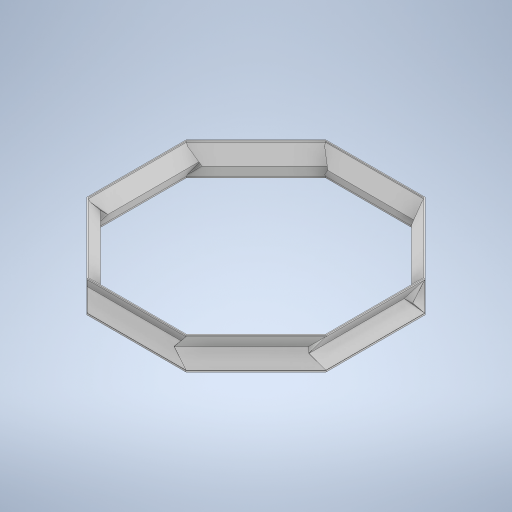
# Autodesk Inventor part: 팔각형 OV-PAM 층 한개
Saved by Autodesk Inventor 2024 (Build 280153000, 153)
## iProperties
Created: 2023-06-16
Part Number: 팔각형 OV-PAM 층 한개
Material: 일반
Document SubType Name: Modeling
Designer: jsw
Density: 1 g/cm^3
Appearance: 기본값
Author: jsw
Autodesk Inventor part; units mm, degrees
ref_plane "YZ Plane" through (0, 0, 0) normal (1, 0, 0) x (0, 1, 0)
ref_plane "XZ Plane" through (0, 0, 0) normal (0, 1, 0) x (-1, 0, 0)
ref_plane "XY Plane" through (0, 0, 0) normal (0, 0, 1) x (1, 0, 0)
sketch "스케치1" plane through (0, 0, 0) normal (0, 1, 0) x (-1, 0, 0)
  line L0 (-97.7756, 40.5) -> (-40.5, 97.7756)
  line L1 (-40.5, 97.7756) -> (40.5, 97.7756)
  line L2 (40.5, 97.7756) -> (97.7756, 40.5)
  line L3 (97.7756, 40.5) -> (97.7756, -40.5)
  line L4 (97.7756, -40.5) -> (40.5, -97.7756)
  line L5 (40.5, -97.7756) -> (-40.5, -97.7756)
  line L6 (-40.5, -97.7756) -> (-97.7756, -40.5)
  line L7 (-97.7756, -40.5) -> (-97.7756, 40.5)
  line L8 (-40.7485, 98.3756) -> (40.7485, 98.3756)
  line L9 (40.7485, 98.3756) -> (98.3756, 40.7485)
  line L10 (98.3756, 40.7485) -> (98.3756, -40.7485)
  line L11 (98.3756, -40.7485) -> (40.7485, -98.3756)
  line L12 (40.7485, -98.3756) -> (-40.7485, -98.3756)
  line L13 (-40.7485, -98.3756) -> (-98.3756, -40.7485)
  line L14 (-98.3756, -40.7485) -> (-98.3756, 40.7485)
  line L15 (-98.3756, 40.7485) -> (-40.7485, 98.3756)
  point P0 (0, 0)
  point P1 (0, 0)
  point P2 (0, 0)
  dimension "d0" = 81
  dimension "d2" = 0.6
  constraints: 32 end point, 2 coincident, 2 horizontal, 34 other
  measures "d0" distance of L0.end L1.end
  measures "d2" distance between parallel lines of L10 L3
extrude "돌출2" add sketch "스케치1" along normal blind 12 contours L0 L1 L2 L3 L4 L5 L6 L7 | L8 L9 L10 L11 L12 L13 L14 L15
ref_plane "작업 평면2" through (98.3756, 0, 40.7485) normal (-0.8660254, -0.5, 0) x (0, 0, -1)
sketch "스케치3" plane through (98.3756, 0, 40.7485) normal (1, 0, 0) x (0, 0, -1)
  line L0 (0, 0) -> (0, 12) projected
  line L1 (0, 12) -> (81.4971, 12) projected
  line L2 (0, 0) -> (81.4971, 0)
  line L3 (81.4971, 0) -> (81.4971, 12)
  line L4 (81.4971, 12) -> (0, 12)
  line L5 (0, 12) -> (0, 0)
  line L6 (0, 12) -> (-7.3047, 12)
  line L7 (-57.6271, 12) -> (0, 12) projected
  line L8 (0, 0) -> (-7.3047, 12)
  line L9 (81.4971, 12) -> (40.7485, 12)
  line L10 (71.4971, 12) -> (81.4971, 0)
  point P0 (40.7485, 0)
  point P1 (71.4971, 12)
  point P2 (40.7485, 12)
  dimension "d17" = 121.33
  dimension "d53" = 10
  constraints: 16 end point, 5 midpoint, 2 parallel, 2 point on line, 1 horizontal, 1 perpendicular
  measures "d17" angle of L8 L2
  measures "d53" distance of L1.end L10.start
extrude "돌출4" cut sketch "스케치3" against normal up to surface contours L8 L6 L0 | L0 L1 L10 L2 surface through (98.3756, 0, 40.7485) normal (-0.8660254, -0.5, 0)
pattern_circular "원형 패턴1" count 8 over 360 about axis through (0, -10, 0) along (0, 1, 0) of "돌출4"
mirror "미러5" about plane through (0, 12, 0) normal (0, 1, 0) of "돌출2", "돌출4", "원형 패턴1"
sketch "스케치9" plane through (-40.7485, 24, -98.3756) normal (0, 1, 0) x (1, 0, 0)
  line L0 (139.1242, -139.1242) -> (139.1242, -57.6271) projected
  line L1 (139.1242, -57.6271) -> (81.4971, 0) projected
  line L2 (81.4971, 0) -> (0, 0) projected
  line L3 (0, 0) -> (-57.6271, -57.6271) projected
  line L4 (-57.6271, -57.6271) -> (-57.6271, -139.1242) projected
  line L5 (-57.6271, -139.1242) -> (0, -196.7513) projected
  line L6 (0, -196.7513) -> (81.4971, -196.7513) projected
  line L7 (81.4971, -196.7513) -> (139.1242, -139.1242) projected
  point P0 (40.7485, -98.3756)
extrude "돌출8" add sketch "스케치9" along normal blind 1.2
sketch "스케치10" plane through (0, 0, 0) normal (0, -1, 0) x (1, 0, 0)
  line L0 (98.3756, 40.7485) -> (98.3756, -40.7485) projected
  line L1 (40.7485, 98.3756) -> (98.3756, 40.7485) projected
  line L2 (-40.7485, 98.3756) -> (40.7485, 98.3756) projected
  line L3 (-98.3756, 40.7485) -> (-40.7485, 98.3756) projected
  line L4 (-98.3756, -40.7485) -> (-98.3756, 40.7485) projected
  line L5 (-40.7485, -98.3756) -> (-98.3756, -40.7485) projected
  line L6 (40.7485, -98.3756) -> (-40.7485, -98.3756) projected
  line L7 (98.3756, -40.7485) -> (40.7485, -98.3756) projected
  point P0 (0, 0)
extrude "돌출9" add sketch "스케치10" along normal blind 1.2
shell "쉘6" thickness 0.6 removed faces 2 at (-13.5828, 25.2, 32.7919) at (13.5828, -1.2, 32.7919)
sketch "스케치12" plane through (-40.7485, 25.2, -98.3756) normal (0, 1, 0) x (1, 0, 0)
  line L0 (138.5242, -57.8756) -> (138.5242, -138.8756) projected
  line L1 (138.5242, -138.8756) -> (81.2485, -196.1513) projected
  line L2 (81.2485, -196.1513) -> (0.2485, -196.1513) projected
  line L3 (0.2485, -196.1513) -> (-57.0271, -138.8756) projected
  line L4 (-57.0271, -138.8756) -> (-57.0271, -57.8756) projected
  line L5 (-57.0271, -57.8756) -> (0.2485, -0.6) projected
  line L6 (0.2485, -0.6) -> (81.2485, -0.6) projected
  line L7 (81.2485, -0.6) -> (138.5242, -57.8756) projected
  line L8 (139.1242, -57.6271) -> (81.4971, 0) projected
  line L9 (81.4971, 0) -> (0, 0) projected
  line L10 (0, 0) -> (-57.6271, -57.6271) projected
  line L11 (-57.6271, -57.6271) -> (-57.6271, -139.1242) projected
  line L12 (-57.6271, -139.1242) -> (0, -196.7513) projected
  line L13 (0, -196.7513) -> (81.4971, -196.7513) projected
  line L14 (81.4971, -196.7513) -> (139.1242, -139.1242) projected
  line L15 (139.1242, -139.1242) -> (139.1242, -57.6271) projected
  line L16 (-0.0828, 0.2) -> (81.5799, 0.2)
  line L17 (81.5799, 0.2) -> (139.3242, -57.5443)
  line L18 (139.3242, -57.5443) -> (139.3242, -139.207)
  line L19 (139.3242, -139.207) -> (81.5799, -196.9513)
  line L20 (81.5799, -196.9513) -> (-0.0828, -196.9513)
  line L21 (-0.0828, -196.9513) -> (-57.8271, -139.207)
  line L22 (-57.8271, -139.207) -> (-57.8271, -57.5443)
  line L23 (-57.8271, -57.5443) -> (-0.0828, 0.2)
  point P0 (40.7485, -98.3756)
  point P1 (40.7485, -98.3756)
  dimension "d50" = 0.2
  constraints: 16 end point, 1 coincident, 1 horizontal, 17 other
  measures "d50" distance between parallel lines of L9 L16
extrude "돌출10" add sketch "스케치12" against normal blind 1.2 contours L16 L17 L18 L19 L20 L21 L22 L23
ref_plane "작업 평면6" through (-40.7485, 12, -98.3756) normal (0, 1, 0) x (1, 0, 0)
mirror "미러8" about plane through (-40.7485, 12, -98.3756) normal (0, 1, 0) of "돌출10"
